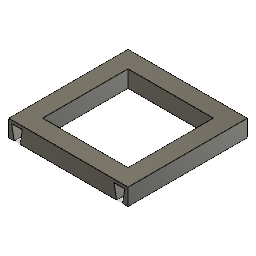
impossible cube (lid~recovered) (Autodesk Fusion 360 design; units mm, degrees)
Autodesk Fusion 360 part; units mm, degrees
sketch "Sketch1" plane through (0, 0, 0) normal (0, 1, 0) x (1, 0, 0)
  line L0 (7.1636, -5.106) -> (96.0636, -5.106)
  line L1 (96.0636, -5.106) -> (96.0636, -94.006)
  line L2 (96.0636, -94.006) -> (7.1636, -94.006)
  line L3 (7.1636, -94.006) -> (7.1636, -5.106)
  line L4 (19.8636, -17.806) -> (83.3636, -17.806)
  line L5 (83.3636, -17.806) -> (83.3636, -81.306)
  line L6 (83.3636, -81.306) -> (19.8636, -81.306)
  line L7 (19.8636, -81.306) -> (19.8636, -17.806)
  dimension "d1" = 88.9
  dimension "d2" = 88.9
  dimension "d3" = 12.7
  dimension "d4" = 12.7
  dimension "d5" = 12.7
  dimension "d6" = 12.7
  constraint horizontal L0
  constraint vertical L1
  constraint horizontal L2
  constraint vertical L3
  constraint horizontal L4
  constraint vertical L5
  constraint horizontal L6
  constraint vertical L7
  measures "d1" distance of L1 L3
  measures "d2" distance of L0.end L1.end
  measures "d3" distance of L0 L4
  measures "d4" distance of L1 L5
  measures "d5" distance of L2 L6
  measures "d6" distance of L3 L7
extrude "Extrude1" add sketch "Sketch1" along normal blind 12.7
sketch "Sketch2" plane through (0, 0, 94.006) normal (0, 0, 1) x (1, 0, 0)
  line L0 (7.1636, 0) -> (96.0636, 0)
  line L1 (96.0636, 0) -> (96.0636, 12.7)
  line L2 (96.0636, 12.7) -> (7.1636, 12.7)
  line L3 (7.1636, 12.7) -> (7.1636, 0)
  line L4 (7.1636, 0) -> (11.4086, 0)
  line L5 (7.1636, 12.7) -> (9.5036, 12.7)
  line L6 (9.5036, 12.7) -> (9.5036, 10.36) construction
  line L7 (7.1636, 0) -> (19.8636, 0)
  line L8 (19.8636, 0) -> (15.6186, 0)
  line L9 (19.8636, 0) -> (19.8636, 12.7) construction
  line L10 (19.8636, 12.7) -> (19.8636, 10.36) construction
  line L11 (19.8636, 10.36) -> (17.5236, 10.36) construction
  line L12 (11.4086, 0) -> (9.5036, 10.36)
  line L13 (9.5036, 10.36) -> (17.5236, 10.36)
  line L14 (15.6186, 0) -> (17.5236, 10.36)
  line L15 (96.0636, 0) -> (83.3636, 0) construction
  line L16 (83.3636, 0) -> (83.3636, 12.7) construction
  line L17 (83.3636, 0) -> (87.6086, 0)
  line L18 (96.0636, 0) -> (91.8186, 0)
  line L19 (83.3636, 12.7) -> (85.7036, 12.7)
  line L20 (85.7036, 12.7) -> (85.7036, 10.36) construction
  line L21 (96.0636, 12.7) -> (93.7236, 12.7)
  line L22 (93.7236, 12.7) -> (93.7236, 10.36) construction
  line L23 (87.6086, 0) -> (85.7036, 10.36)
  line L24 (85.7036, 10.36) -> (93.7236, 10.36)
  line L25 (93.7236, 10.36) -> (91.8186, 0)
  dimension "d9" = 4.245
  dimension "d10" = 2.34
  dimension "d11" = 2.34
  dimension "d12" = 12.7
  dimension "d13" = 4.245
  dimension "d14" = 2.34
  dimension "d15" = 2.34
  dimension "d16" = 12.7
  dimension "d17" = 12.7
  dimension "d18" = 4.245
  dimension "d19" = 4.245
  dimension "d20" = 2.34
  dimension "d21" = 2.34
  dimension "d22" = 2.34
  dimension "d23" = 2.34
  constraint coincident L0.start L3.end
  constraint perpendicular L3 L4
  constraint coincident L2.end L3.start
  constraint perpendicular L3 L5
  constraint perpendicular L5 L6
  constraint perpendicular L3 L7
  constraint parallel L0 L8
  constraint coincident L2 L9.end
  constraint perpendicular L2 L9
  constraint perpendicular L2 L10
  constraint perpendicular L9 L11
  constraint coincident L0.end L1.start
  constraint perpendicular L1 L15
  constraint perpendicular L2 L16
  constraint perpendicular L16 L17
  constraint perpendicular L1 L18
  constraint perpendicular L16 L19
  constraint perpendicular L2 L20
  constraint coincident L1.end L2.start
  constraint perpendicular L1 L21
  constraint perpendicular L21 L22
  measures "d9" distance of L0.start L4.end
  measures "d10" distance of L2.end L5.end
  measures "d11" distance of L5.end L6.end
  measures "d12" distance of L0.start L7.end
  measures "d13" distance of L7.end L8.end
  measures "d14" distance of L9.end L10.end
  measures "d15" distance of L10.end L11.end
  measures "d16" distance of L0.end L15.end
  measures "d17" distance of L15.end L16.end
  measures "d18" distance of L15.end L17.end
  measures "d19" distance of L0.end L18.end
  measures "d20" distance of L16.end L19.end
  measures "d21" distance of L19.end L20.end
  measures "d22" distance of L1.end L21.end
  measures "d23" distance of L21.end L22.end
extrude "Extrude2" cut sketch "Sketch2" against normal blind 88.9 contours L0 L7 L12 L13 L14 | L0 L23 L24 L25
equation "d11 = 0.1 in - 0.2 mm"
equation "d13 = 0.175 in - 0.2 mm"
